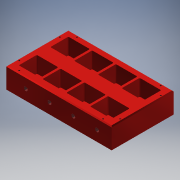
# Autodesk Inventor part: UNLHEP-14-01-P-004_ChuckForGantry
Saved by Autodesk Inventor 2019.4 (Build 234330000, 330)
## iProperties
Created: 2014-01-09
Part Number: UNLHEP-14-01-P-004_ChuckForGantry
Material: Aluminum, Anodized Red
Document SubType Name: Modeling
Designer: Frank Meier
Density: 2.7 g/cm^3
Project: UNL Pixel Phase I
Mass: 2699.72 g
Surface Area: 1115.91 cm^2
Volume: 999.896 cm^3
Appearance: Anodized - Red
Author: Frank Meier
Revision Number: 00
Autodesk Inventor part; units mm, degrees
ref_plane "YZ Plane" through (0, 0, 0) normal (1, 0, 0) x (0, 1, 0)
ref_plane "XZ Plane" through (0, 0, 0) normal (0, 1, 0) x (-1, 0, 0)
ref_plane "XY Plane" through (0, 0, 0) normal (0, 0, 1) x (1, 0, 0)
sketch "Skizze1" plane through (0, 0, 0) normal (0, 0, 1) x (1, 0, 0)
  line L0 (-117, -69) -> (117, -69)
  line L1 (117, -69) -> (117, 69)
  line L2 (117, 69) -> (-117, 69)
  line L3 (-117, 69) -> (-117, -69)
  line L4 (-117, -69) -> (117, 69) construction
  line L5 (117, -69) -> (-117, 69) construction
  point P0 (0, 0)
  dimension "d0" = 234
  dimension "d2" = 138
  constraints: 12 end point, 2 midpoint, 2 parallel, 1 horizontal, 1 perpendicular
  measures "d0" distance of L1.end L2.end
  measures "d2" distance of L0.end L1.end
extrude "Extrusion1" add sketch "Skizze1" along normal blind 46
chamfer "Fase1" distance 2 angle 45 4 edges at (0, -69, 46) (-117, 0, 46) (0, 69, 46) (117, 0, 46)
sketch "Skizze4" plane through (0, 0, 46) normal (0, 0, 1) x (1, 0, 0)
  line L0 (117, 69) -> (-117, 69) projected
  line L1 (117, -69) -> (117, 69) projected
  line L2 (-117, 69) -> (-117, -69) projected
  line L3 (-117, -69) -> (117, -69) projected
  point P0 (-112, 45)
  point P1 (-112, -45)
  point P2 (-93, -64)
  point P3 (-93, 64)
  point P4 (93, 64)
  point P5 (112, 45)
  point P6 (112, -45)
  point P7 (93, -64)
  dimension "d153" = 24
  dimension "d154" = 24
  dimension "d155" = 5
  dimension "d156" = 5
  dimension "d157" = 24
  dimension "d158" = 5
  dimension "d159" = 5
  dimension "d160" = 24
  dimension "d161" = 24
  dimension "d162" = 5
  dimension "d163" = 5
  dimension "d164" = 24
  dimension "d165" = 5
  dimension "d166" = 24
  dimension "d167" = 5
  dimension "d168" = 24
  measures "d153" distance from line of L0 point (-112, 45)
  measures "d154" distance from line of L3 point (-112, -45)
  measures "d155" distance from line of L2 point (-112, -45)
  measures "d156" distance from line of L3 point (-93, -64)
  measures "d157" distance from line of L2 point (-93, -64)
  measures "d158" distance from line of L2 point (-112, 45)
  measures "d159" distance from line of L0 point (-93, 64)
  measures "d160" distance from line of L2 point (-93, 64)
  measures "d161" distance from line of L1 point (93, 64)
  measures "d162" distance from line of L0 point (93, 64)
  measures "d163" distance from line of L1 point (112, 45)
  measures "d164" distance from line of L0 point (112, 45)
  measures "d165" distance from line of L1 point (112, -45)
  measures "d166" distance from line of L3 point (112, -45)
  measures "d167" distance from line of L3 point (93, -64)
  measures "d168" distance from line of L1 point (93, -64)
hole "Bohrung7" at (-112, 45, 46) at (-112, -45, 46) at (-93, -64, 46) at (-93, 64, 46) at (93, 64, 46) at (112, 45, 46) at (112, -45, 46) at (93, -64, 46) direction (0, 0, -1) diameter 3.242 depth 20 tip angle 118 thread size "M4x0.7" class "6H" standard "ISO Metric profile"
sketch "Sketch12" plane through (0, 0, 46) normal (0, 0, 1) x (1, 0, 0)
  line L0 (-101.5, 55.5) -> (-57.75, 55.5)
  line L1 (-55.75, 53.5) -> (-55.75, 17.5)
  line L2 (-57.75, 15.5) -> (-101.5, 15.5)
  line L3 (-103.5, 17.5) -> (-103.5, 53.5)
  circle A0 centre (-112, 45) radius 1.621 projected
  circle A1 centre (-112, 45) radius 1.621 projected
  circle A2 centre (-93, 64) radius 1.621 projected
  arc A3 (-101.5, 55.5) -> (-103.5, 53.5) centre (-101.5, 53.5) ccw
  arc A4 (-55.75, 53.5) -> (-57.75, 55.5) centre (-57.75, 53.5) ccw
  arc A5 (-57.75, 15.5) -> (-55.75, 17.5) centre (-57.75, 17.5) ccw
  arc A6 (-103.5, 17.5) -> (-101.5, 15.5) centre (-101.5, 17.5) ccw
  arc A7 (-48.75, 55.5) -> (-50.75, 53.5) centre (-48.75, 53.5) ccw
  line L4 (-50.75, 17.5) -> (-50.75, 53.5)
  line L5 (-48.75, 55.5) -> (-5, 55.5)
  arc A8 (-3, 53.5) -> (-5, 55.5) centre (-5, 53.5) ccw
  line L6 (-3, 53.5) -> (-3, 17.5)
  arc A9 (-5, 15.5) -> (-3, 17.5) centre (-5, 17.5) ccw
  line L7 (-5, 15.5) -> (-48.75, 15.5)
  arc A10 (-50.75, 17.5) -> (-48.75, 15.5) centre (-48.75, 17.5) ccw
  arc A11 (4, 55.5) -> (2, 53.5) centre (4, 53.5) ccw
  line L8 (2, 17.5) -> (2, 53.5)
  line L9 (4, 55.5) -> (47.75, 55.5)
  arc A12 (49.75, 53.5) -> (47.75, 55.5) centre (47.75, 53.5) ccw
  line L10 (49.75, 53.5) -> (49.75, 17.5)
  arc A13 (47.75, 15.5) -> (49.75, 17.5) centre (47.75, 17.5) ccw
  line L11 (47.75, 15.5) -> (4, 15.5)
  arc A14 (2, 17.5) -> (4, 15.5) centre (4, 17.5) ccw
  arc A15 (56.75, 55.5) -> (54.75, 53.5) centre (56.75, 53.5) ccw
  line L12 (54.75, 17.5) -> (54.75, 53.5)
  line L13 (56.75, 55.5) -> (100.5, 55.5)
  arc A16 (102.5, 53.5) -> (100.5, 55.5) centre (100.5, 53.5) ccw
  line L14 (102.5, 53.5) -> (102.5, 17.5)
  arc A17 (100.5, 15.5) -> (102.5, 17.5) centre (100.5, 17.5) ccw
  line L15 (100.5, 15.5) -> (56.75, 15.5)
  arc A18 (54.75, 17.5) -> (56.75, 15.5) centre (56.75, 17.5) ccw
  arc A19 (-101.5, -14.5) -> (-103.5, -16.5) centre (-101.5, -16.5) ccw
  line L16 (-103.5, -52.5) -> (-103.5, -16.5)
  line L17 (-101.5, -14.5) -> (-57.75, -14.5)
  arc A20 (-55.75, -16.5) -> (-57.75, -14.5) centre (-57.75, -16.5) ccw
  line L18 (-55.75, -16.5) -> (-55.75, -52.5)
  arc A21 (-57.75, -54.5) -> (-55.75, -52.5) centre (-57.75, -52.5) ccw
  line L19 (-57.75, -54.5) -> (-101.5, -54.5)
  arc A22 (-103.5, -52.5) -> (-101.5, -54.5) centre (-101.5, -52.5) ccw
  arc A23 (-48.75, -14.5) -> (-50.75, -16.5) centre (-48.75, -16.5) ccw
  line L20 (-50.75, -52.5) -> (-50.75, -16.5)
  line L21 (-48.75, -14.5) -> (-5, -14.5)
  arc A24 (-3, -16.5) -> (-5, -14.5) centre (-5, -16.5) ccw
  line L22 (-3, -16.5) -> (-3, -52.5)
  arc A25 (-5, -54.5) -> (-3, -52.5) centre (-5, -52.5) ccw
  line L23 (-5, -54.5) -> (-48.75, -54.5)
  arc A26 (-50.75, -52.5) -> (-48.75, -54.5) centre (-48.75, -52.5) ccw
  arc A27 (4, -14.5) -> (2, -16.5) centre (4, -16.5) ccw
  line L24 (2, -52.5) -> (2, -16.5)
  line L25 (4, -14.5) -> (47.75, -14.5)
  arc A28 (49.75, -16.5) -> (47.75, -14.5) centre (47.75, -16.5) ccw
  line L26 (49.75, -16.5) -> (49.75, -52.5)
  arc A29 (47.75, -54.5) -> (49.75, -52.5) centre (47.75, -52.5) ccw
  line L27 (47.75, -54.5) -> (4, -54.5)
  arc A30 (2, -52.5) -> (4, -54.5) centre (4, -52.5) ccw
  arc A31 (56.75, -14.5) -> (54.75, -16.5) centre (56.75, -16.5) ccw
  line L28 (54.75, -52.5) -> (54.75, -16.5)
  line L29 (56.75, -14.5) -> (100.5, -14.5)
  arc A32 (102.5, -16.5) -> (100.5, -14.5) centre (100.5, -16.5) ccw
  line L30 (102.5, -16.5) -> (102.5, -52.5)
  arc A33 (100.5, -54.5) -> (102.5, -52.5) centre (100.5, -52.5) ccw
  line L31 (100.5, -54.5) -> (56.75, -54.5)
  arc A34 (54.75, -52.5) -> (56.75, -54.5) centre (56.75, -52.5) ccw
  point P0 (0, 0)
  point P1 (-55.75, 15.5)
  point P2 (-55.75, 55.5)
  point P3 (-103.5, 15.5)
  point P4 (-50.75, 15.5)
  point P5 (-3, 55.5)
  point P6 (-3, 15.5)
  point P7 (2, 15.5)
  point P8 (49.75, 55.5)
  point P9 (49.75, 15.5)
  point P10 (54.75, 15.5)
  point P11 (102.5, 55.5)
  point P12 (102.5, 15.5)
  point P13 (-103.5, -54.5)
  point P14 (-55.75, -14.5)
  point P15 (-55.75, -54.5)
  point P16 (-50.75, -54.5)
  point P17 (-3, -14.5)
  point P18 (-3, -54.5)
  point P19 (2, -54.5)
  point P20 (49.75, -14.5)
  point P21 (49.75, -54.5)
  point P22 (54.75, -54.5)
  point P23 (102.5, -14.5)
  point P24 (102.5, -54.5)
  dimension "d193" = 47.75
  dimension "d194" = 40
  dimension "d195" = 8.5
  dimension "d196" = 8.5
  dimension "d197" = 2
  dimension "d200" = 52.75
  dimension "d203" = 70
  constraints: 64 end point, 64 point on circle, 48 point on line, 32 centre point, 8 tangent, 3 equal radius, 2 collinear, 2 horizontal, 2 parallel, 1 perpendicular, 1 vertical, 159 other
  measures "d193" distance of point (-55.75, 15.5) point (-103.5, 15.5)
  measures "d194" distance of point (-55.75, 55.5) point (-55.75, 15.5)
  measures "d195" distance from line of L3 point (-112, 45)
  measures "d196" distance from line of L0 point (-93, 64)
  measures "d197" radius of A3
  measures "d200" distance of L3.end L4.end
  measures "d203" distance of L3.end L16.end
extrude "Extrusion5" cut sketch "Sketch12" against normal blind 36 contours L0 A4 L1 A5 L2 A6 L3 A3 | L5 A8 L6 A9 L7 A10 L4 A7 | L9 A12 L10 A13 L11 A14 L8 A11 | L13 A16 L14 A17 L15 A18 L12 A15 | L17 A20 L18 A21 L19 A22 L16 A19 | L21 A24 L22 A25 L23 A26 L20 A23 | L25 A28 L26 A29 L27 A30 L24 A27 | L29 A32 L30 A33 L31 A34 L28 A31
sketch "Sketch13" plane through (-117, -69, 0) normal (0, -1, 0) x (1, 0, 0)
  line L0 (232, 46) -> (2, 46) projected
  point P0 (117, 0)
  point P1 (43.375, 23)
  point P2 (96.125, 23)
  point P3 (148.875, 23)
  point P4 (201.625, 23)
  dimension "d209" = 23
  dimension "d212" = 52.75
  constraints: 1 horizontal, 3 other
  measures "d209" distance from line of point (43.375, 23) L0
  measures "d212" distance of point (43.375, 23) point (96.125, 23)
hole "Hole9" at (-73.625, -69, 23) at (-20.875, -69, 23) at (31.875, -69, 23) at (84.625, -69, 23) direction (0, 1, 0) diameter 7.95 depth 14.5 tip angle 118 taper from width 8.7366 to width 8.304 over 6.924 thread size "1/8" designation "1/8 - 27 NPT" standard "NPT"
sketch "Sketch14" plane through (-117, 69, 0) normal (0, 1, 0) x (1, 0, 0)
  circle A0 centre (43.375, -23) radius 4.3684 projected
  line L0 (234, -44) -> (0, -44) projected
  point P0 (117, 0)
  point P1 (43.375, -23)
  point P2 (96.125, -23)
  point P3 (148.875, -23)
  point P4 (201.625, -23)
  dimension "d228" = 52.75
  constraints: 1 coincident, 1 horizontal, 3 other
  measures "d228" distance of point (43.375, -23) point (96.125, -23)
hole "Hole10" at (-73.625, 69, 23) at (-20.875, 69, 23) at (31.875, 69, 23) at (84.625, 69, 23) direction (0, -1, 0) diameter 7.95 depth 13.5 tip angle 118 taper from width 8.7366 to width 8.304 over 6.924 thread size "1/8" designation "1/8 - 27 NPT" standard "NPT"
sketch "Sketch15" plane through (0, 0, 0) normal (0, 0, -1) x (-1, 0, 0)
  line L0 (117, -69) -> (-117, -69) projected
  line L1 (117, 69) -> (117, -69) projected
  point P0 (0, 0)
  point P1 (25, -25)
  point P2 (-25, -25)
  point P3 (25, 25)
  point P4 (-25, 25)
  dimension "d242" = 25
  dimension "d243" = 25
  dimension "d246" = 50
  dimension "d249" = 50
  constraints: 1 horizontal, 1 vertical, 3 other
  measures "d242" horizontal distance of point (0, 0) point (25, -25)
  measures "d243" horizontal distance of point (0, 0) point (25, -25)
  measures "d246" distance of point (25, -25) point (-25, -25)
  measures "d249" distance of point (25, -25) point (25, 25)
hole "Hole11" at (-25, -25, 0) at (25, -25, 0) at (-25, 25, 0) at (25, 25, 0) direction (0, 0, 1) diameter 6.756 depth 10 tip angle 118 clearance for "Flat Head Machine Screw (82)" size "1/4" standard "Ansi Unified Screw Threads"
